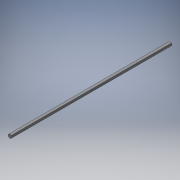
# Autodesk Inventor part: hex shaft 1
Saved by Autodesk Inventor 2018 (Build 220112000, 112)
## iProperties
Created: 2020-01-22
Part Number: hex shaft 1
Material: Generic
Document SubType Name: Modeling
Designer: s-2513225
Density: 1 g/cm^3
Appearance: Default
Author: s-2513225
Autodesk Inventor part; units mm, degrees
ref_plane "YZ Plane" through (0, 0, 0) normal (1, 0, 0) x (0, 1, 0)
ref_plane "XZ Plane" through (0, 0, 0) normal (0, 1, 0) x (-1, 0, 0)
ref_plane "XY Plane" through (0, 0, 0) normal (0, 0, 1) x (1, 0, 0)
sketch "Sketch1" plane through (0, 0, 0) normal (0, 0, 1) x (1, 0, 0)
  line L0 (7.111, -1.7879) -> (2.0072, -7.0523)
  line L1 (2.0072, -7.0523) -> (-5.1039, -5.2644)
  line L2 (-5.1039, -5.2644) -> (-7.111, 1.7879)
  line L3 (-7.111, 1.7879) -> (-2.0072, 7.0523)
  line L4 (-2.0072, 7.0523) -> (5.1039, 5.2644)
  line L5 (5.1039, 5.2644) -> (7.111, -1.7879)
  point P0 (0, 0)
  point P1 (0, 0)
  point P2 (0, 0)
  dimension "d3" = 12.7
  constraints: 12 end point, 2 coincident, 13 other
  measures "d3" distance between parallel lines of L1 L4
extrude "Extrusion1" add sketch "Sketch1" along normal blind 355.6
body "Solid1"
